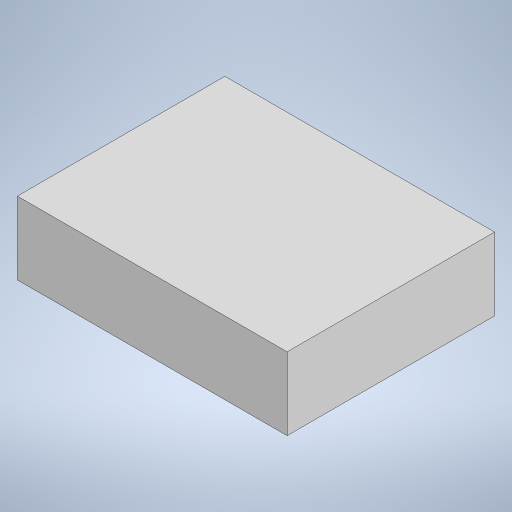
# Autodesk Inventor part: Repeat Dual - Temp
Saved by Autodesk Inventor 2023.4 (Build 274418000, 418)
## iProperties
Created: 2024-05-11
Part Number: Repeat Dual - Temp
Material: Generic
Document SubType Name: Modeling
Designer: Nathan Cai
Density: 1.64835 g/cm^3
Appearance: Default
Mass: 6 g
Surface Area: 16.84 cm^2
Volume: 3.64 cm^3
Author: Nathan Cai
Autodesk Inventor part; units mm, degrees
ref_plane "YZ Plane" through (0, 0, 0) normal (1, 0, 0) x (0, 1, 0)
ref_plane "XZ Plane" through (0, 0, 0) normal (0, 1, 0) x (-1, 0, 0)
ref_plane "XY Plane" through (0, 0, 0) normal (0, 0, 1) x (1, 0, 0)
sketch "Sketch1" plane through (0, 0, 0) normal (0, 1, 0) x (-1, 0, 0)
  line L0 (-13, 10) -> (13, 10)
  line L1 (13, 10) -> (13, -10)
  line L2 (13, -10) -> (-13, -10)
  line L3 (-13, -10) -> (-13, 10)
  line L4 (-13, 10) -> (13, -10) construction
  line L5 (13, 10) -> (-13, -10) construction
  point P0 (0, 0)
  dimension "d0" = 26
  dimension "d1" = 20
  constraints: 12 end point, 2 midpoint, 2 parallel, 1 horizontal, 1 perpendicular
  measures "d0" distance of L1.end L2.end
  measures "d1" distance of L0.end L1.end
extrude "Extrusion1" add sketch "Sketch1" along normal blind 7
body "Solid1"
